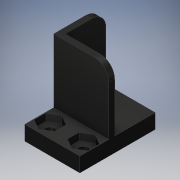
# Autodesk Inventor part: EquerreBatterieGauche
Saved by Autodesk Inventor 2019 (Build 230136000, 136)
## iProperties
Created: 2019-07-30
Part Number: EquerreBatterieGauche
Material: Plastique ABS
Document SubType Name: Modeling
Designer: Sébastien DI MERCURIO
Mass: 14.1383 g
Surface Area: 34.18 cm^2
Volume: 13.338 cm^3
Density: 1.06 g/cm^3
Appearance: Lustré - Noir
Author: Sébastien DI MERCURIO
Autodesk Inventor part; units mm, degrees
ref_plane "YZ Plane" through (0, 0, 0) normal (1, 0, 0) x (0, 1, 0)
ref_plane "XZ Plane" through (0, 0, 0) normal (0, 1, 0) x (-1, 0, 0)
ref_plane "XY Plane" through (0, 0, 0) normal (0, 0, 1) x (1, 0, 0)
sketch "Esquisse1" plane through (0, 0, 0) normal (0, 0, 1) x (1, 0, 0)
  line L0 (0, 0) -> (19, 0)
  line L1 (19, 0) -> (19, 27)
  line L2 (19, 27) -> (0, 27)
  line L3 (0, 27) -> (0, 0)
  dimension "d0" = 27
  dimension "d1" = 19
  constraints: 8 end point, 2 parallel, 1 horizontal, 1 perpendicular
  measures "d0" distance of L0.end L1.end
  measures "d1" distance of L0.start L0.end
extrude "Extrusion1" add sketch "Esquisse1" along normal blind 26
sketch "Esquisse2" plane through (0, 27, 0) normal (0, 1, 0) x (1, 0, 0)
  line L0 (19, 0) -> (2, 0)
  line L1 (2, 0) -> (2, -14)
  line L2 (2, -14) -> (19, -14)
  line L3 (19, -14) -> (19, 0)
  line L4 (0, 0) -> (0, -26) projected
  line L5 (19, 0) -> (19, -26) projected
  line L6 (0, -26) -> (19, -26)
  line L7 (19, -26) -> (19, -16)
  line L8 (19, -16) -> (0, -16)
  line L9 (0, -16) -> (0, -26)
  dimension "d4" = 2
  dimension "d5" = 2
  dimension "d6" = 14
  dimension "d7" = 10
  constraints: 16 end point, 4 parallel, 2 horizontal, 2 perpendicular, 1 point on line
  measures "d4" distance between parallel lines of L4 L1
  measures "d5" distance between parallel lines of L8 L2
  measures "d6" distance between parallel lines of L2 L0
  measures "d7" distance between parallel lines of L6 L8
extrude "Extrusion2" cut sketch "Esquisse2" against normal blind 22
sketch "Esquisse3" plane through (0, 5, 0) normal (0, 1, 0) x (1, 0, 0)
  circle A0 centre (3.75, -21) radius 1.5
  circle A1 centre (15.25, -21) radius 1.5
  line L0 (0, -16) -> (19, -16) projected
  line L1 (19, -16) -> (19, -26) projected
  line L2 (0, -26) -> (0, -16) projected
  point P0 (0, 0)
  dimension "d10" = 3
  dimension "d11" = 5
  dimension "d12" = 11.5
  dimension "d13" = 19
  dimension "d14" = 3.75
  constraints: 2 centre point, 1 equal radius, 1 horizontal alignment
  measures "d10" diameter of A0
  measures "d11" distance from line of A0.centre L0
  measures "d12" distance of A1.centre A0.centre
  measures "d13" distance between parallel lines of L1 L2
  measures "d14" distance from line of L2 A0.centre
extrude "Extrusion3" cut sketch "Esquisse3" against normal through all
sketch "Esquisse4" plane through (0, 5, 0) normal (0, 1, 0) x (1, 0, 0)
  circle A0 centre (3.75, -21) radius 1.5 projected
  line L0 (3.75, -16.9585) -> (7.25, -18.9793)
  line L1 (7.25, -18.9793) -> (7.25, -23.0207)
  line L2 (7.25, -23.0207) -> (3.75, -25.0415)
  line L3 (3.75, -25.0415) -> (0.25, -23.0207)
  line L4 (0.25, -23.0207) -> (0.25, -18.9793)
  line L5 (0.25, -18.9793) -> (3.75, -16.9585)
  circle A1 centre (15.25, -21) radius 1.5 projected
  line L6 (15.25, -16.9585) -> (18.75, -18.9793)
  line L7 (18.75, -18.9793) -> (18.75, -23.0207)
  line L8 (18.75, -23.0207) -> (15.25, -25.0415)
  line L9 (15.25, -25.0415) -> (11.75, -23.0207)
  line L10 (11.75, -23.0207) -> (11.75, -18.9793)
  line L11 (11.75, -18.9793) -> (15.25, -16.9585)
  point P0 (0, 0)
  dimension "d17" = 7
  constraints: 24 end point, 2 coincident, 2 vertical alignment, 1 parallel, 26 other
  measures "d17" distance between parallel lines of L2 L5
extrude "Extrusion4" cut sketch "Esquisse4" against normal blind 2.5
fillet "Congé1" radius 5 2 edges at (1, 27, 0) (19, 27, 15)
equation "\"d14\" = -0.5 * d12 + 0.5 * d13"
